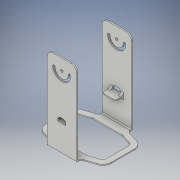
# Autodesk Inventor part: AR.Drone2.0
Saved by Autodesk Inventor 2019 (Build 230136000, 136)
## iProperties
Created: 2020-01-23
Part Number: AR.Drone2.0
Material: Generic
Document SubType Name: Modeling
Designer: Next
Density: 1 g/cm^3
Appearance: Default
Author: Next
Autodesk Inventor part; units mm, degrees
ref_plane "YZ Plane" through (0, 0, 0) normal (1, 0, 0) x (0, 1, 0)
ref_plane "XZ Plane" through (0, 0, 0) normal (0, 1, 0) x (-1, 0, 0)
ref_plane "XY Plane" through (0, 0, 0) normal (0, 0, 1) x (1, 0, 0)
sketch "Sketch1" plane through (0, 0, 0) normal (0, 1, 0) x (-1, 0, 0)
  line L0 (0, 0) -> (-140, 0) construction
  line L1 (-140, 0) -> (-140, -100) construction
  line L2 (-140, -100) -> (0, -100) construction
  line L3 (0, -100) -> (0, 0) construction
  line L4 (0, -50) -> (-140, -50) construction
  line L5 (-70, -100) -> (-70, 0) construction
  line L6 (-96.6886, -17.5) -> (-43.3114, -17.5) construction
  line L7 (-120, -71.3962) -> (-120, -28.6038) construction
  line L8 (-20, -28.6038) -> (-20, -71.3962) construction
  line L9 (-98.2698, -82.2434) -> (-116.5811, -76.1396)
  line L10 (-116.5811, -23.8604) -> (-98.2698, -17.7566)
  line L11 (-41.7302, -17.7566) -> (-23.4189, -23.8604)
  line L12 (-23.4189, -76.1396) -> (-41.7302, -82.2434)
  line L13 (-43.3114, -82.5) -> (-96.6886, -82.5)
  arc A0 (-23.4189, -76.1396) -> (-20, -71.3962) centre (-25, -71.3962) ccw
  arc A1 (-43.3114, -82.5) -> (-41.7302, -82.2434) centre (-43.3114, -77.5) ccw
  arc A2 (-98.2698, -82.2434) -> (-96.6886, -82.5) centre (-96.6886, -77.5) ccw
  arc A3 (-120, -71.3962) -> (-116.5811, -76.1396) centre (-115, -71.3962) ccw
  arc A4 (-116.5811, -23.8604) -> (-120, -28.6038) centre (-115, -28.6038) ccw
  arc A5 (-96.6886, -17.5) -> (-98.2698, -17.7566) centre (-96.6886, -22.5) ccw
  arc A6 (-41.7302, -17.7566) -> (-43.3114, -17.5) centre (-43.3114, -22.5) ccw
  arc A7 (-20, -28.6038) -> (-23.4189, -23.8604) centre (-25, -28.6038) ccw
  line L14 (-120, -71.3962) -> (-120, -28.6038)
  line L15 (-20, -28.6038) -> (-20, -71.3962)
  arc A8 (-101.432, -91.7302) -> (-100.4386, -92.0237) centre (-96.6886, -77.5) ccw
  line L16 (-101.432, -91.7302) -> (-119.7434, -85.6265)
  arc A9 (-130, -71.3962) -> (-119.7434, -85.6265) centre (-115, -71.3962) ccw
  line L17 (-130, -71.3962) -> (-130, -28.6038)
  arc A10 (-119.7434, -14.3735) -> (-130, -28.6038) centre (-115, -28.6038) ccw
  line L18 (-119.7434, -14.3735) -> (-101.432, -8.2698)
  arc A11 (-100.4386, -7.9763) -> (-101.432, -8.2698) centre (-96.6886, -22.5) ccw
  arc A12 (-38.568, -8.2698) -> (-39.5614, -7.9763) centre (-43.3114, -22.5) ccw
  line L19 (-38.568, -8.2698) -> (-20.2566, -14.3735)
  arc A13 (-10, -28.6038) -> (-20.2566, -14.3735) centre (-25, -28.6038) ccw
  line L20 (-10, -28.6038) -> (-10, -71.3962)
  arc A14 (-20.2566, -85.6265) -> (-10, -71.3962) centre (-25, -71.3962) ccw
  line L21 (-20.2566, -85.6265) -> (-38.568, -91.7302)
  arc A15 (-39.5614, -92.0237) -> (-38.568, -91.7302) centre (-43.3114, -77.5) ccw
  line L22 (-96.6886, -17.5) -> (-43.3114, -17.5)
  line L23 (-96.6886, -3.1351) -> (-96.6886, 1.5)
  line L24 (-96.6886, 1.5) -> (-43.3114, 1.5)
  line L25 (-43.3114, 1.5) -> (-43.3114, -3.1351)
  line L26 (-96.6886, -96.8649) -> (-96.6886, -101.5)
  line L27 (-96.6886, -101.5) -> (-43.3114, -101.5)
  line L28 (-43.3114, -101.5) -> (-43.3114, -96.8649)
  arc A16 (-96.6886, -96.8649) -> (-100.4386, -92.0237) centre (-101.6886, -96.8649) ccw
  arc A17 (-39.5614, -92.0237) -> (-43.3114, -96.8649) centre (-38.3114, -96.8649) ccw
  arc A18 (-43.3114, -3.1351) -> (-39.5614, -7.9763) centre (-38.3114, -3.1351) ccw
  arc A19 (-100.4386, -7.9763) -> (-96.6886, -3.1351) centre (-101.6886, -3.1351) ccw
  point P0 (-70, -50)
  dimension "d41" = 5
  dimension "d0" = 140
  dimension "d1" = 100
  dimension "d6" = 5
  dimension "d10" = 5
  constraints: 58 end point, 40 point on circle, 23 tangent, 20 centre point, 10 equal radius, 10 parallel, 5 midpoint, 3 horizontal, 2 perpendicular, 12 other
  measures "d0" distance of L2.end L1.end
  measures "d1" distance of L1.end L0.end
  measures "d6" radius of A0
  measures "d10" radius of A16
extrude "Extrusion1" add sketch "Sketch1" along normal blind 2
sketch "Sketch2" plane through (0, 2, 0) normal (0, 1, 0) x (1, 0, 0)
  line L0 (43.3114, 1) -> (96.6886, 1) construction
  line L1 (43.3114, 99) -> (96.6886, 99) construction
  line L2 (96.6886, 101.5) -> (43.3114, 101.5) construction
  line L3 (43.3114, -1.5) -> (96.6886, -1.5) construction
  line L4 (43.3114, -1.5) -> (96.6886, -1.5) projected
  line L5 (43.3114, 1) -> (96.6886, 1)
  line L6 (96.6886, 1) -> (96.6886, -1.5)
  line L7 (96.6886, -1.5) -> (43.3114, -1.5)
  line L8 (43.3114, -1.5) -> (43.3114, 1)
  line L9 (43.3114, 101.5) -> (96.6886, 101.5)
  line L10 (96.6886, 101.5) -> (96.6886, 99)
  line L11 (96.6886, 99) -> (43.3114, 99)
  line L12 (43.3114, 99) -> (43.3114, 101.5)
  point P0 (0, 0)
  dimension "d13" = 2.5
  dimension "d14" = 2.5
  constraints: 20 end point, 4 horizontal, 4 parallel, 2 perpendicular
  measures "d13" distance between parallel lines of L1 L2
  measures "d14" distance between parallel lines of L3 L0
extrude "Extrusion2" add sketch "Sketch2" along normal blind 150
fillet "Fillet1" radius 2 4 edges at (70, 2, -1) (70, 2, -99) (70, 0, 1.5) (70, 0, -101.5)
sketch "Sketch3" plane through (96.6886, 0, -101.5) normal (0, 0, -1) x (-1, 0, 0)
  line L0 (0, 2) -> (0, 152) construction
  line L1 (0, 132) -> (24.3997, 132) construction
  line L2 (0, 152) -> (53.3772, 152) construction
  circle A0 centre (26.6497, 132) radius 2.25
  line L3 (28.8997, 132) -> (53.2994, 132) construction
  line L4 (24.3997, 132) -> (28.8997, 132) construction
  circle A1 centre (41.0995, 132) radius 2.25
  circle A2 centre (12.1998, 132) radius 2.25
  arc A3 (9.9498, 132) -> (43.3495, 132) centre (26.6497, 132) ccw
  arc A4 (14.4498, 132) -> (38.8495, 132) centre (26.6497, 132) ccw
  arc A5 (14.4498, 132) -> (9.9498, 132) centre (12.1998, 132) ccw
  arc A6 (43.3495, 132) -> (38.8495, 132) centre (41.0995, 132) ccw
  point P0 (96.6886, 0)
  point P1 (0, 0)
  dimension "d19" = 4.5
  dimension "d20" = 4.5
  dimension "d21" = 4.5
  dimension "d42" = 4.5
  constraints: 10 point on circle, 7 centre point, 6 end point, 4 tangent, 3 horizontal, 2 midpoint, 1 point on line
  measures "d19" diameter of A0
  measures "d20" diameter of A1
  measures "d21" diameter of A2
  measures "d42" diameter of A6
extrude "Extrusion3" cut sketch "Sketch3" against normal blind 110
fillet "Fillet2" radius 10 4 edges at (43.3114, 152, -100.25) (96.6886, 152, -100.25) (43.3114, 152, 0.25) (96.6886, 152, 0.25)
sketch "Sketch4" plane through (96.6886, 0, -101.5) normal (0, 0, -1) x (-1, 0, 0)
  line L0 (0, 2) -> (53.3772, 2) construction
  line L1 (34.1886, 49) -> (19.1886, 49)
  line L2 (19.1886, 49) -> (19.1886, 57)
  line L3 (19.1886, 57) -> (34.1886, 57)
  line L4 (34.1886, 57) -> (34.1886, 49)
  point P0 (96.6886, 0)
  dimension "d26" = 15
  dimension "d27" = 8
  dimension "d28" = 47
  constraints: 8 end point, 2 parallel, 1 horizontal, 1 perpendicular
  measures "d26" distance of L2.end L3.end
  measures "d27" distance of L1.end L2.end
  measures "d28" distance between parallel lines of L1 L0
extrude "Extrusion4" cut sketch "Sketch4" against normal blind 110
fillet "Fillet3" radius 5 4 edges at (62.5, 57, -100.25) (77.5, 57, -100.25) (62.5, 57, 0.25) (77.5, 57, 0.25)
sketch "Sketch5" plane through (96.6886, 4, -1) normal (0, 0, -1) x (-1, 0, 0)
  line L0 (39.1886, 45) -> (14.1886, 45)
  line L1 (14.1886, 45) -> (14.1886, 43)
  line L2 (14.1886, 43) -> (39.1886, 43)
  line L3 (39.1886, 43) -> (39.1886, 45)
  line L4 (34.1886, 45) -> (19.1886, 45) projected
  point P0 (96.6886, -4)
  point P1 (26.6886, 44)
  dimension "d32" = 25
  dimension "d33" = 2
  constraints: 8 end point, 2 parallel, 1 horizontal, 1 perpendicular, 1 other
  measures "d32" distance of L2.end L1.end
  measures "d33" distance of L1.end L0.end
extrude "Extrusion5" add sketch "Sketch5" along normal blind 98
sketch "Sketch6" plane through (62.5, 49, -101.5) normal (0, 1, 0) x (1, 0, 0)
  line L0 (-5, -17.5) -> (20, -17.5)
  line L1 (20, -17.5) -> (20, -85.5)
  line L2 (20, -85.5) -> (-5, -85.5)
  line L3 (-5, -85.5) -> (-5, -17.5)
  line L4 (20, -100.5) -> (15, -100.5) construction
  line L5 (0, -100.5) -> (-5, -100.5) construction
  line L6 (20, -100.5) -> (-5, -100.5) construction
  line L7 (15, -2.5) -> (20, -2.5) construction
  line L8 (-5, -2.5) -> (0, -2.5) construction
  line L9 (20, -2.5) -> (-5, -2.5) construction
  point P0 (-62.5, -101.5)
  dimension "d37" = 15
  dimension "d38" = 15
  constraints: 12 end point, 2 horizontal, 2 parallel, 1 collinear, 1 perpendicular
  measures "d37" distance between parallel lines of L2 L6
  measures "d38" distance between parallel lines of L9 L0
extrude "Extrusion6" cut sketch "Sketch6" against normal blind 3
fillet "Fillet4" radius 5 10 edges at (70, 47, -1) (70, 47, -99) (80, 49, -99) (60, 49, -99) (80, 49, -1) (60, 49, -1) (82.5, 48, -16) (57.5, 48, -16) (82.5, 48, -84) (57.5, 48, -84)
body "Solid1"
